Autodesk Inventor part; units mm, degrees
(part 2 of 2)
  line L413 (10.425, 23.6738) -> (10.425, 23.9738)
  line L414 (10.0988, 23.9738) -> (10.0988, 23.6738)
  line L415 (10.175, 23.9738) -> (10.0988, 23.9738)
  line L416 (10.0988, 23.6738) -> (10.175, 23.6738)
  line L417 (10.175, 23.6738) -> (10.175, 23.9738)
  line L418 (9.8488, 23.9738) -> (9.8488, 23.6738)
  line L419 (9.925, 23.9738) -> (9.8488, 23.9738)
  line L420 (9.8488, 23.6738) -> (9.925, 23.6738)
  line L421 (9.925, 23.6738) -> (9.925, 23.9738)
  line L422 (9.5988, 23.9738) -> (9.5988, 23.6738)
  line L423 (9.675, 23.9738) -> (9.5988, 23.9738)
  line L424 (9.5988, 23.6738) -> (9.675, 23.6738)
  line L425 (9.675, 23.6738) -> (9.675, 23.9738)
  line L426 (9.3488, 23.9738) -> (9.3488, 23.6738)
  line L427 (9.425, 23.9738) -> (9.3488, 23.9738)
  line L428 (9.3488, 23.6738) -> (9.425, 23.6738)
  line L429 (9.425, 23.6738) -> (9.425, 23.9738)
  line L430 (9.0988, 23.9738) -> (9.0988, 23.6738)
  line L431 (9.175, 23.9738) -> (9.0988, 23.9738)
  line L432 (9.0988, 23.6738) -> (9.175, 23.6738)
  line L433 (9.175, 23.6738) -> (9.175, 23.9738)
  line L434 (8.8488, 23.9738) -> (8.8488, 23.6738)
  line L435 (8.925, 23.9738) -> (8.8488, 23.9738)
  line L436 (8.8488, 23.6738) -> (8.925, 23.6738)
  line L437 (8.925, 23.6738) -> (8.925, 23.9738)
  line L438 (8.5988, 23.9738) -> (8.5988, 23.6738)
  line L439 (8.675, 23.9738) -> (8.5988, 23.9738)
  line L440 (8.5988, 23.6738) -> (8.675, 23.6738)
  line L441 (8.675, 23.6738) -> (8.675, 23.9738)
  line L442 (8.3488, 23.9738) -> (8.3488, 23.6738)
  line L443 (8.425, 23.9738) -> (8.3488, 23.9738)
  line L444 (8.3488, 23.6738) -> (8.425, 23.6738)
  line L445 (8.425, 23.6738) -> (8.425, 23.9738)
  line L446 (8.0988, 23.9738) -> (8.0988, 23.6738)
  line L447 (8.175, 23.9738) -> (8.0988, 23.9738)
  line L448 (8.0988, 23.6738) -> (8.175, 23.6738)
  line L449 (8.175, 23.6738) -> (8.175, 23.9738)
  line L450 (7.8488, 23.9738) -> (7.8488, 23.6738)
  line L451 (7.925, 23.9738) -> (7.8488, 23.9738)
  line L452 (7.8488, 23.6738) -> (7.925, 23.6738)
  line L453 (7.925, 23.6738) -> (7.925, 23.9738)
  line L454 (7.5988, 23.9738) -> (7.5988, 23.6738)
  line L455 (7.675, 23.9738) -> (7.5988, 23.9738)
  line L456 (7.5988, 23.6738) -> (7.675, 23.6738)
  line L457 (7.675, 23.6738) -> (7.675, 23.9738)
  line L458 (7.3488, 23.9738) -> (7.3488, 23.6738)
  line L459 (7.425, 23.9738) -> (7.3488, 23.9738)
  line L460 (7.3488, 23.6738) -> (7.425, 23.6738)
  line L461 (7.425, 23.6738) -> (7.425, 23.9738)
  line L462 (7.0988, 23.9738) -> (7.0988, 23.6738)
  line L463 (7.175, 23.9738) -> (7.0988, 23.9738)
  line L464 (7.0988, 23.6738) -> (7.175, 23.6738)
  line L465 (7.175, 23.6738) -> (7.175, 23.9738)
  line L466 (6.8488, 23.9738) -> (6.8488, 23.6738)
  line L467 (6.925, 23.9738) -> (6.8488, 23.9738)
  line L468 (6.8488, 23.6738) -> (6.925, 23.6738)
  line L469 (6.925, 23.6738) -> (6.925, 23.9738)
  line L470 (6.5988, 23.9738) -> (6.5988, 23.6738)
  line L471 (6.675, 23.9738) -> (6.5988, 23.9738)
  line L472 (6.5988, 23.6738) -> (6.675, 23.6738)
  line L473 (6.675, 23.6738) -> (6.675, 23.9738)
  line L474 (6.3488, 23.9738) -> (6.3488, 23.6738)
  line L475 (6.425, 23.9738) -> (6.3488, 23.9738)
  line L476 (6.3488, 23.6738) -> (6.425, 23.6738)
  line L477 (6.425, 23.6738) -> (6.425, 23.9738)
  line L478 (6.0988, 23.9738) -> (6.0988, 23.6738)
  line L479 (6.175, 23.9738) -> (6.0988, 23.9738)
  line L480 (6.0988, 23.6738) -> (6.175, 23.6738)
  line L481 (6.175, 23.6738) -> (6.175, 23.9738)
  line L482 (5.8488, 23.9738) -> (5.8488, 23.6738)
  line L483 (5.925, 23.9738) -> (5.8488, 23.9738)
  line L484 (5.8488, 23.6738) -> (5.925, 23.6738)
  line L485 (5.925, 23.6738) -> (5.925, 23.9738)
  line L486 (5.5988, 23.9738) -> (5.5988, 23.6738)
  line L487 (5.675, 23.9738) -> (5.5988, 23.9738)
  line L488 (5.5988, 23.6738) -> (5.675, 23.6738)
  line L489 (5.675, 23.6738) -> (5.675, 23.9738)
  line L490 (5.3488, 23.9738) -> (5.3488, 23.6738)
  line L491 (5.425, 23.9738) -> (5.3488, 23.9738)
  line L492 (5.3488, 23.6738) -> (5.425, 23.6738)
  line L493 (5.425, 23.6738) -> (5.425, 23.9738)
  line L494 (5.0988, 23.9738) -> (5.0988, 23.6738)
  line L495 (5.175, 23.9738) -> (5.0988, 23.9738)
  line L496 (5.0988, 23.6738) -> (5.175, 23.6738)
  line L497 (5.175, 23.6738) -> (5.175, 23.9738)
  line L498 (4.8488, 23.9738) -> (4.8488, 23.6738)
  line L499 (4.925, 23.9738) -> (4.8488, 23.9738)
  line L500 (4.8488, 23.6738) -> (4.925, 23.6738)
  line L501 (4.925, 23.6738) -> (4.925, 23.9738)
  line L502 (4.5988, 23.9738) -> (4.5988, 23.6738)
  line L503 (4.675, 23.9738) -> (4.5988, 23.9738)
  line L504 (4.5988, 23.6738) -> (4.675, 23.6738)
  line L505 (4.675, 23.6738) -> (4.675, 23.9738)
  line L506 (4.3488, 23.9738) -> (4.3488, 23.6738)
  line L507 (4.425, 23.9738) -> (4.3488, 23.9738)
  line L508 (4.3488, 23.6738) -> (4.425, 23.6738)
  line L509 (4.425, 23.6738) -> (4.425, 23.9738)
  line L510 (4.0988, 23.9738) -> (4.0988, 23.6738)
  line L511 (4.175, 23.9738) -> (4.0988, 23.9738)
  line L512 (4.0988, 23.6738) -> (4.175, 23.6738)
  line L513 (4.175, 23.6738) -> (4.175, 23.9738)
  line L514 (3.8488, 23.9738) -> (3.8488, 23.6738)
  line L515 (3.925, 23.9738) -> (3.8488, 23.9738)
  line L516 (3.8488, 23.6738) -> (3.925, 23.6738)
  line L517 (3.925, 23.6738) -> (3.925, 23.9738)
  line L518 (3.5988, 23.9738) -> (3.5988, 23.6738)
  line L519 (3.675, 23.9738) -> (3.5988, 23.9738)
  line L520 (3.5988, 23.6738) -> (3.675, 23.6738)
  line L521 (3.675, 23.6738) -> (3.675, 23.9738)
  line L522 (3.3488, 23.9738) -> (3.3488, 23.6738)
  line L523 (3.425, 23.9738) -> (3.3488, 23.9738)
  line L524 (3.3488, 23.6738) -> (3.425, 23.6738)
  line L525 (3.425, 23.6738) -> (3.425, 23.9738)
  line L526 (3.0988, 23.9738) -> (3.0988, 23.6738)
  line L527 (3.175, 23.9738) -> (3.0988, 23.9738)
  line L528 (3.0988, 23.6738) -> (3.175, 23.6738)
  line L529 (3.175, 23.6738) -> (3.175, 23.9738)
  line L530 (2.8488, 23.9738) -> (2.8488, 23.6738)
  line L531 (2.925, 23.9738) -> (2.8488, 23.9738)
  line L532 (2.8488, 23.6738) -> (2.925, 23.6738)
  line L533 (2.925, 23.6738) -> (2.925, 23.9738)
  line L534 (2.5988, 23.9738) -> (2.5988, 23.6738)
  line L535 (2.675, 23.9738) -> (2.5988, 23.9738)
  line L536 (2.5988, 23.6738) -> (2.675, 23.6738)
  line L537 (2.675, 23.6738) -> (2.675, 23.9738)
  line L538 (2.3488, 23.9738) -> (2.3488, 23.6738)
  line L539 (2.425, 23.9738) -> (2.3488, 23.9738)
  line L540 (2.3488, 23.6738) -> (2.425, 23.6738)
  line L541 (2.425, 23.6738) -> (2.425, 23.9738)
  line L542 (2.0988, 23.9738) -> (2.0988, 23.6738)
  line L543 (2.175, 23.9738) -> (2.0988, 23.9738)
  line L544 (2.0988, 23.6738) -> (2.175, 23.6738)
  line L545 (2.175, 23.6738) -> (2.175, 23.9738)
  line L546 (1.8488, 23.9738) -> (1.8488, 23.6738)
  line L547 (1.925, 23.9738) -> (1.8488, 23.9738)
  line L548 (1.8488, 23.6738) -> (1.925, 23.6738)
  line L549 (1.925, 23.6738) -> (1.925, 23.9738)
  line L550 (1.5988, 23.9738) -> (1.5988, 23.6738)
  line L551 (1.675, 23.9738) -> (1.5988, 23.9738)
  line L552 (1.5988, 23.6738) -> (1.675, 23.6738)
  line L553 (1.675, 23.6738) -> (1.675, 23.9738)
  line L554 (1.3488, 23.9738) -> (1.3488, 23.6738)
  line L555 (1.425, 23.9738) -> (1.3488, 23.9738)
  line L556 (1.3488, 23.6738) -> (1.425, 23.6738)
  line L557 (1.425, 23.6738) -> (1.425, 23.9738)
  line L558 (1.0988, 23.9738) -> (1.0988, 23.6738)
  line L559 (1.175, 23.9738) -> (1.0988, 23.9738)
  line L560 (1.0988, 23.6738) -> (1.175, 23.6738)
  line L561 (1.175, 23.6738) -> (1.175, 23.9738)
  line L562 (0.8488, 23.9738) -> (0.8488, 23.6738)
  line L563 (0.925, 23.9738) -> (0.8488, 23.9738)
  line L564 (0.8488, 23.6738) -> (0.925, 23.6738)
  line L565 (0.925, 23.6738) -> (0.925, 23.9738)
  line L566 (0.5988, 23.9738) -> (0.5988, 23.6738)
  line L567 (0.675, 23.9738) -> (0.5988, 23.9738)
  line L568 (0.5988, 23.6738) -> (0.675, 23.6738)
  line L569 (0.675, 23.6738) -> (0.675, 23.9738)
  point P0 (0, 0)
  dimension "d57" = 0.0762
  dimension "d58" = 0.3
  dimension "d59" = 3
  dimension "d60" = 3.9
  dimension "d63" = 0.25
  dimension "d68" = 0.3
  dimension "d69" = 0.0762
  dimension "d70" = 0.125
  dimension "d71" = 0.0762
  dimension "d74" = 0.25
  constraints: 1136 end point, 4 horizontal, 4 parallel, 2 perpendicular, 1120 other
  measures "d57" distance of L2.end L1.end
  measures "d58" distance of L1.end L0.end
  measures "d59" distance between parallel lines of L4 L3
  measures "d60" distance between parallel lines of L5 L0
  measures "d63" distance of L0.start L6.start
  measures "d68" distance of L288.end L286.start
  measures "d69" distance of L287.end L288.end
  measures "d70" distance between parallel lines of L289 L3
  measures "d71" distance between parallel lines of L286 L2
  measures "d74" distance of L287.end L290.end
extrude "Extrusion4" add sketch "Sketch8" along normal blind 0.05
equation "\"d35\" = 0.5 * d33"
equation "\"d36\" = 0.5 * d34"
equation "\"d68\" = d58"
equation "\"d69\" = d57"
equation "\"d70\" = 0.5 * d63"
body "Solid1"
